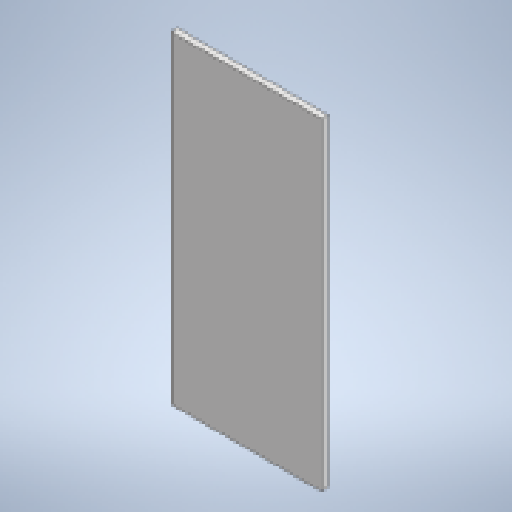
# Autodesk Inventor part: Tapa
Saved by Autodesk Inventor 2024 (Build 280153000, 153)
## iProperties
Created: 2025-05-11
Part Number: Tapa
Material: Genérico
Document SubType Name: Modeling
Designer: sergi
Density: 1 g/cm^3
Appearance: Valor por defecto
Author: sergi
Autodesk Inventor part; units mm, degrees
ref_plane "YZ Plane" through (0, 0, 0) normal (1, 0, 0) x (0, 1, 0)
ref_plane "XZ Plane" through (0, 0, 0) normal (0, 1, 0) x (-1, 0, 0)
ref_plane "XY Plane" through (0, 0, 0) normal (0, 0, 1) x (1, 0, 0)
sketch "Boceto1" plane through (0, 0, 0) normal (0, 0, 1) x (1, 0, 0)
  line L0 (-15.5, -18.5) -> (-17.5, -18.5) projected
  line L1 (-17.5, -18.5) -> (-17.5, -37.5) projected
  line L2 (-17.5, -37.5) -> (17.5, -37.5) projected
  line L3 (17.5, -37.5) -> (17.5, 37.5) projected
  line L4 (17.5, 37.5) -> (-17.5, 37.5) projected
  line L5 (-17.5, 37.5) -> (-17.5, -0.5) projected
  line L6 (-17.5, -0.5) -> (-15.5, -0.5) projected
  line L7 (-15.5, -0.5) -> (-15.5, 35.5) projected
  line L8 (-15.5, 35.5) -> (15.5, 35.5) projected
  line L9 (15.5, 35.5) -> (15.5, -35.5) projected
  line L10 (15.5, -35.5) -> (-15.5, -35.5) projected
  line L11 (-15.5, -35.5) -> (-15.5, -18.5) projected
  line L12 (15.5, 35.5) -> (-15.5, 35.5)
  line L13 (-15.5, 35.5) -> (-15.5, -35.5)
  line L14 (-15.5, -35.5) -> (15.5, -35.5)
  line L15 (15.5, -35.5) -> (15.5, 35.5)
  line L16 (-15.3, -35.3) -> (-15.3, 35.3)
  line L17 (-15.3, 35.3) -> (15.3, 35.3)
  line L18 (15.3, 35.3) -> (15.3, -35.3)
  line L19 (15.3, -35.3) -> (-15.3, -35.3)
  line L20 (-14.1, 34.1) -> (-14.1, -34.1)
  line L21 (-14.1, -34.1) -> (14.1, -34.1)
  line L22 (14.1, -34.1) -> (14.1, 34.1)
  line L23 (14.1, 34.1) -> (-14.1, 34.1)
  line L24 (-15.5, -0.5) -> (-14.1, -0.5)
  line L25 (-15.5, -18.5) -> (-14.1, -18.5)
  point P0 (0, 0)
  point P1 (-15.3, -0.5)
  point P2 (-15.3, -18.5)
  dimension "d0" = 0.2
  dimension "d1" = 1.2
  constraints: 28 end point, 6 parallel, 5 perpendicular, 2 point on line, 1 horizontal, 6 other
  measures "d0" distance between parallel lines of L13 L16
  measures "d1" distance between parallel lines of L16 L20
extrude "Extrusión1" add sketch "Boceto1" against normal blind 3 contours L25 L20 L21 L22 L23 L24 L16 L17 L18 L19
chamfer "Chaflán1" distance 0.8 angle 45 5 edges at (-15.3, 17.4, -3) (-15.3, -26.9, -3) (0, -35.3, -3) (15.3, 0, -3) (0, 35.3, -3)
sketch "Boceto2" plane through (0, 0, 0) normal (0, 0, 1) x (1, 0, 0)
  line L0 (-15.5, -18.5) -> (-17.5, -18.5) projected
  line L1 (-17.5, -18.5) -> (-17.5, -37.5) projected
  line L2 (-17.5, -37.5) -> (17.5, -37.5) projected
  line L3 (17.5, -37.5) -> (17.5, 37.5) projected
  line L4 (17.5, 37.5) -> (-17.5, 37.5) projected
  line L5 (-17.5, 37.5) -> (-17.5, -0.5) projected
  line L6 (-17.5, -0.5) -> (-15.5, -0.5) projected
  line L7 (-15.5, -0.5) -> (-15.5, 35.5) projected
  line L8 (-15.5, 35.5) -> (15.5, 35.5) projected
  line L9 (15.5, 35.5) -> (15.5, -35.5) projected
  line L10 (15.5, -35.5) -> (-15.5, -35.5) projected
  line L11 (-15.5, -35.5) -> (-15.5, -18.5) projected
  line L12 (-17.5, -0.5) -> (-17.5, -18.5)
  point P0 (0, 0)
  constraints: 2 end point, 1 vertical
extrude "Extrusión2" add sketch "Boceto2" along normal blind 1.5
sketch "Boceto3" plane through (0, 0, 1.5) normal (0, 0, 1) x (1, 0, 0)
  line L0 (-17.5, 37.5) -> (-17.5, -37.5) projected
  line L1 (-17.5, -37.5) -> (17.5, -37.5) projected
  line L2 (17.5, -37.5) -> (17.5, 37.5) projected
  line L3 (17.5, 37.5) -> (-17.5, 37.5) projected
  line L4 (-15.5, 35.5) -> (15.5, 35.5) projected
  line L5 (-15.5, -35.5) -> (-15.5, 35.5) projected
  line L6 (15.5, -35.5) -> (-15.5, -35.5) projected
  line L7 (15.5, 35.5) -> (15.5, -35.5) projected
  line L8 (-15.5, 35.5) -> (-15.5, 15.5)
  line L9 (-15.5, 15.5) -> (-0.5, 15.5)
  line L10 (-0.5, 15.5) -> (-15.5, 15.5)
  line L11 (-15.5, 15.5) -> (-15.5, 0.5)
  line L12 (-15.5, 0.5) -> (-0.5, 0.5)
  line L13 (-0.5, 0.5) -> (-0.5, 15.5)
  circle A0 centre (-8, 8) radius 7.5
  point P0 (0, 0)
  dimension "d9" = 20
  dimension "d11" = 15
  dimension "d12" = 15
  dimension "d13" = 15
  constraints: 12 end point, 3 tangent, 2 horizontal, 2 parallel, 1 centre point, 1 perpendicular, 1 point on line
  measures "d9" distance of L4.start L8.end
  measures "d11" distance of L8.end L9.end
  measures "d12" distance of L12.end L11.end
  measures "d13" distance of L12.end L9.end
extrude "Extrusión3" cut sketch "Boceto3" against normal through all contours A0
